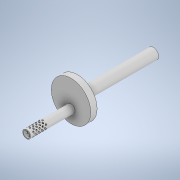
# Autodesk Inventor part: Eccentric_Shaft
Saved by Autodesk Inventor 2021 (Build 250183000, 183)
## iProperties
Created: 2021-03-26
Part Number: Eccentric_Shaft
Material: Generic
Document SubType Name: Modeling
Designer: lucia
Density: 1 g/cm^3
Appearance: Default
Author: lucia
Autodesk Inventor part; units mm, degrees
ref_plane "YZ Plane" through (0, 0, 0) normal (1, 0, 0) x (0, 1, 0)
ref_plane "XZ Plane" through (0, 0, 0) normal (0, 1, 0) x (-1, 0, 0)
ref_plane "XY Plane" through (0, 0, 0) normal (0, 0, 1) x (1, 0, 0)
sketch "Sketch1" plane through (0, 0, 0) normal (0, 0, 1) x (1, 0, 0)
  circle A0 centre (0, 0) radius 10.668
  dimension "d0" = 21.336
  constraints: 1 centre point, 1 coincident
  measures "d0" diameter of A0
extrude "Extrusion1" add sketch "Sketch1" against normal blind 152.4
sketch "Sketch2" plane through (0, 0, 0) normal (0, 0, 1) x (1, 0, 0)
  circle A0 centre (0, 0) radius 39.624
  dimension "d3" = 79.248
  constraints: 1 centre point, 1 coincident
  measures "d3" diameter of A0
extrude "Extrusion2" add sketch "Sketch2" along normal blind 12.7
sketch "Sketch3" plane through (0, 0, 12.7) normal (0, 0, 1) x (1, 0, 0)
  circle A0 centre (0, -13.208) radius 8.128
  line L0 (0, 0) -> (0, -13.208)
  dimension "d6" = 16.256
  dimension "d7" = 13.208
  constraints: 2 end point, 1 centre point, 1 vertical
  measures "d6" diameter of A0
  measures "d7" distance of L0.start L0.end
extrude "Extrusion3" add sketch "Sketch3" along normal blind 88.9
sketch "Sketch10" plane through (0, -13.208, 101.6) normal (0, 0, 1) x (1, 0, 0)
  circle A0 centre (0, 0) radius 6.5405
  point P0 (0, 13.208)
  dimension "d27" = 13.081
  constraints: 1 centre point
  measures "d27" diameter of A0
extrude "Extrusion6" cut sketch "Sketch10" against normal blind 34.798
sketch "Sketch11" plane through (0, -13.208, 101.6) normal (0, 0, 1) x (1, 0, 0)
  circle A0 centre (0, 0) radius 6.5405
  circle A1 centre (0, 0) radius 8.128
  point P0 (0, 13.208)
  dimension "d30" = 13.081
  dimension "d31" = 16.256
  constraints: 2 centre point, 1 coincident
  measures "d30" diameter of A0
  measures "d31" diameter of A1
ref_plane "Work Plane2" through (0, -13.208, 12.7) normal (-1, 0, 0) x (0, 0, 1)
sketch "Sketch12" plane through (0, -13.208, 12.7) normal (-1, 0, 0) x (0, 0, 1)
  line L0 (88.9, -8.128) -> (88.9, 8.128) projected
  line L1 (88.9, 0) -> (101.6, 0)
  line L2 (101.6, 0) -> (114.3, 0) construction
  line L3 (114.3, 0) -> (114.3, 13.208) construction
  line L4 (114.3, 13.208) -> (127, 13.208) construction
  spline S0 degree 3 poles (101.6, 0) (114.3, 0) (114.3, 13.208) (127, 13.208) knots 1 1 1 1 2 2 2 2
  point P0 (-12.7, 13.208)
  dimension "d32" = 12.7
  dimension "d35" = 13.208
  dimension "d36" = 13.208
  dimension "d37" = 25.4
  dimension "d38" = 12.7
  dimension "d39" = 12.7
  constraints: 2 end point, 2 horizontal, 1 midpoint, 3 other
  measures "d32" distance of L1.start L1.end
  measures "d35" vertical distance of L1.end L4.end
  measures "d36" vertical distance of L1.end L3.end
  measures "d37" horizontal distance of L1.end L4.end
  measures "d38" horizontal distance of L1.end L3.end
  measures "d39" distance of L1.end L2.end
sweep "Sweep1" [suppressed]
sketch "Sketch13" plane through (0, 0, 0) normal (0, 1, 0) x (-1, 0, 0)
  line L0 (0, 0) -> (0, 101.6)
  line L1 (8.128, 101.6) -> (-8.128, 101.6) projected
  circle A0 centre (0, 95.25) radius 1.5875
  circle A1 centre (0, 88.9) radius 1.5875
  circle A2 centre (0, 82.55) radius 1.5875
  circle A3 centre (0, 76.2) radius 1.5875
  circle A4 centre (0, 69.85) radius 1.5875
  point P0 (0, 63.5)
  dimension "d42" = 38.1
  dimension "d43" = 3.175
  dimension "d44" = 6.35
  dimension "d45" = 3.175
  dimension "d46" = 3.175
  dimension "d47" = 3.175
  dimension "d48" = 6.35
  dimension "d49" = 6.35
  dimension "d50" = 6.35
  dimension "d51" = 3.175
  dimension "d52" = 6.35
  constraints: 6 point on line, 5 centre point, 2 end point, 1 midpoint
  measures "d42" distance from line of L1 point (0, 63.5)
  measures "d43" diameter of A0
  measures "d44" distance from line of L1 A0.centre
  measures "d45" diameter of A1
  measures "d46" diameter of A2
  measures "d47" diameter of A3
  measures "d48" distance of A0.centre A1.centre
  measures "d49" distance of A1.centre A2.centre
  measures "d50" distance of A2.centre A3.centre
  measures "d51" diameter of A4
  measures "d52" distance of A4.centre A3.centre
extrude "Extrusion7" cut sketch "Sketch13" against normal blind 13.208
pattern_circular "Circular Pattern1" count 6 over 360 about axis through (0, -13.208, 12.7) along (0, 0, 1) of "Extrusion7"
sketch "Sketch14" plane through (0, 0, 0) normal (1, 0, 0) x (0, 1, 0)
  line L0 (0, 0) -> (0, 101.6)
  circle A0 centre (0, 95.25) radius 1.5875
  circle A1 centre (0, 88.9) radius 1.5875
  circle A2 centre (0, 82.55) radius 1.5875
  circle A3 centre (0, 76.2) radius 1.5875
  circle A4 centre (0, 69.85) radius 1.5875
  line L1 (-19.7485, 101.6) -> (-6.6675, 101.6) projected
  line L2 (-13.208, 101.6) -> (-13.208, 0)
  circle A5 centre (-13.208, 92.075) radius 1.5875
  circle A6 centre (-13.208, 85.725) radius 1.5875
  circle A7 centre (-13.208, 79.375) radius 1.5875
  circle A8 centre (-13.208, 73.025) radius 1.5875
  point P0 (0, 63.5)
  dimension "d59" = 3.175
  dimension "d61" = 3.175
  dimension "d62" = 3.175
  dimension "d63" = 3.175
  dimension "d64" = 6.35
  dimension "d65" = 6.35
  dimension "d66" = 6.35
  dimension "d67" = 3.175
  dimension "d68" = 6.35
  dimension "d69" = 3.175
  dimension "d70" = 3.175
  dimension "d71" = 3.175
  dimension "d72" = 3.175
  dimension "d73" = 9.525
  dimension "d74" = 6.35
  dimension "d75" = 6.35
  dimension "d76" = 6.35
  constraints: 10 point on line, 9 centre point, 4 end point, 2 vertical, 1 midpoint
  measures "d59" diameter of A0
  measures "d61" diameter of A1
  measures "d62" diameter of A2
  measures "d63" diameter of A3
  measures "d64" distance of A0.centre A1.centre
  measures "d65" distance of A1.centre A2.centre
  measures "d66" distance of A2.centre A3.centre
  measures "d67" diameter of A4
  measures "d68" distance of A4.centre A3.centre
  measures "d69" diameter of A5
  measures "d70" diameter of A6
  measures "d71" diameter of A7
  measures "d72" diameter of A8
  measures "d73" distance from line of L1 A5.centre
  measures "d74" distance of A5.centre A6.centre
  measures "d75" distance of A7.centre A8.centre
  measures "d76" distance of A6.centre A7.centre
extrude "Extrusion8" cut sketch "Sketch14" against normal blind 13.208 contours A5 L2 | L2 A5 | A6 L2 | L2 A6 | A7 L2 | L2 A7 | A8 L2 | L2 A8
pattern_circular "Circular Pattern2" count 6 over 360 about axis through (0, -13.208, 12.7) along (0, 0, 1) of "Extrusion8"
equation "\"d1\" = 38.1 * scale"
equation "\"d3\" = 19.812 * scale"
equation "\"d4\" = 3.175 * scale"
equation "\"d6\" = 4.064 * scale"
equation "\"d7\" = 3.302 * scale"
equation "\"d8\" = 22.225 * scale"
equation "\"d35\" = 3.302 * scale"
equation "\"d36\" = 3.302 * scale"
equation "\"d53\" = 3.302 * scale"
equation "\"d77\" = 3.302 * scale"
equation "\"radius\" = 3.175"
equation "\"scale\" = 4"
body "Solid1"
